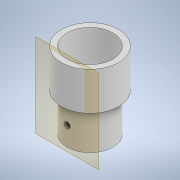
# Autodesk Inventor part: Tube_3
Saved by Autodesk Inventor 2022.3 (Build 263350000, 350)
## iProperties
Created: 2023-03-29
Part Number: Tube_3
Material: Generic
Document SubType Name: Modeling
Designer: Manuel Hueso Béjar
Density: 1 g/cm^3
Appearance: Default
Author: Manuel Hueso Béjar
Autodesk Inventor part; units mm, degrees
ref_plane "YZ Plane" through (0, 0, 0) normal (1, 0, 0) x (0, 1, 0)
ref_plane "XZ Plane" through (0, 0, 0) normal (0, 1, 0) x (-1, 0, 0)
sketch "Sketch1" plane through (0, 0, 0) normal (0, 1, 0) x (-1, 0, 0)
  circle A0 centre (0, 0) radius 12
  circle A1 centre (0, 0) radius 15
  dimension "d0" = 24
  dimension "d1" = 30
  constraints: 2 centre point, 2 coincident
  measures "d0" diameter of A0
  measures "d1" diameter of A1
extrude "Extrusion1" add sketch "Sketch1" against normal blind 20 contours A0
extrude "Extrusion2" add sketch "Sketch1" along normal blind 20
ref_plane "Work Plane1" through (0, 0, 12) normal (0, 0, 1) x (1, 0, 0)
sketch "Sketch2" plane through (0, 0, 12) normal (0, 0, 1) x (1, 0, 0)
  line L0 (-12, -20) -> (12, -20) projected
  line L1 (0, -20) -> (0, 0)
  line L2 (0, -10) -> (-5, -10)
  dimension "d7" = 5
  constraints: 4 end point, 2 midpoint, 1 horizontal, 1 vertical
  measures "d7" distance of L2.start L2.end
hole "Hole1" at (0, -10, 12) direction (0, 0, -1) diameter 2.2 depth 5.8 counterbore diameter 3.1 counterbore depth 4.6
mirror "Mirror1" about plane through (0, 0, 0) normal (0, 0, 1) of "Hole1"
body "Solid1"
